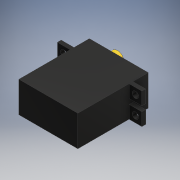
# Autodesk Inventor part: microservo_FT_2322
Saved by Autodesk Inventor 2018 (Build 220112000, 112)
## iProperties
Created: 2018-04-24
Part Number: microservo_FT_2322
Material: Genérico
Document SubType Name: Modeling
Designer: se_ma
Density: 1 g/cm^3
Appearance: Valor por defecto
Author: se_ma
Autodesk Inventor part; units mm, degrees
ref_plane "YZ Plane" through (0, 0, 0) normal (1, 0, 0) x (0, 1, 0)
ref_plane "XZ Plane" through (0, 0, 0) normal (0, 1, 0) x (-1, 0, 0)
ref_plane "XY Plane" through (0, 0, 0) normal (0, 0, 1) x (1, 0, 0)
sketch "Boceto1" plane through (0, 0, 0) normal (0, 1, 0) x (-1, 0, 0)
  line L0 (0, 0) -> (23, 0)
  line L1 (23, 0) -> (23, -12)
  line L2 (23, -12) -> (0, -12)
  line L3 (0, -12) -> (0, 0)
  dimension "d0" = 23
  dimension "d1" = 12
  constraints: 8 end point, 2 parallel, 1 horizontal, 1 perpendicular
  measures "d0" distance of L1.end L2.end
  measures "d1" distance of L0.end L1.end
extrude "Extrusión1" add sketch "Boceto1" along normal blind 27.5
sketch "Boceto2" plane through (0, 27.5, 0) normal (0, 1, 0) x (1, 0, 0)
  line L0 (0, 0) -> (0, 12) projected
  line L1 (0, 0) -> (0, 12)
  line L2 (0, 6) -> (-17, 6)
  circle A0 centre (-17, 6) radius 4.25
  circle A1 centre (-17, 6) radius 2.5
  dimension "d4" = 17
  dimension "d5" = 8.5
  dimension "d6" = 5
  constraints: 4 end point, 2 centre point, 2 coincident, 1 collinear, 1 horizontal, 1 midpoint
  measures "d4" distance of L2.start L2.end
  measures "d5" diameter of A0
  measures "d6" diameter of A1
extrude "Extrusión2" add sketch "Boceto2" along normal blind 5 contours A1
sketch "Boceto3" plane through (0, 27.5, 0) normal (0, 1, 0) x (1, 0, 0)
  circle A0 centre (-17, 6) radius 2.5 projected
  circle A1 centre (-17, 6) radius 4.25
  point P0 (0, 0)
  dimension "d9" = 8.5
  constraints: 1 centre point, 1 coincident
  measures "d9" diameter of A1
extrude "Extrusión3" add sketch "Boceto3" along normal blind 1.5
sketch "Boceto4" plane through (-23, 0, -12) normal (-1, 0, 0) x (0, 0, 1)
  line L0 (12, 0) -> (12, 27.5) projected
  line L1 (12, 27.5) -> (12, 20)
  line L2 (12, 20) -> (12, 21.5)
  line L3 (0, 0) -> (0, 27.5) projected
  line L4 (12, 21.5) -> (7, 21.5)
  line L5 (7, 21.5) -> (7, 20)
  line L6 (7, 20) -> (12, 20)
  line L7 (0, 21.5) -> (5, 21.5)
  line L8 (5, 21.5) -> (5, 20)
  line L9 (5, 20) -> (0, 20)
  line L10 (0, 21.5) -> (0, 20)
  dimension "d12" = 7.5
  dimension "d13" = 1.5
  dimension "d14" = 5
  dimension "d15" = 5
  constraints: 18 end point, 8 point on line, 3 perpendicular, 1 collinear, 1 horizontal
  measures "d12" distance of L0.end L1.end
  measures "d13" distance of L1.end L2.end
  measures "d14" distance of L2.end L4.end
  measures "d15" distance of L7.start L7.end
extrude "Extrusión4" add sketch "Boceto4" along normal blind 5 and the other way blind 28
sketch "Boceto5" plane through (-23, 21.5, -7) normal (0, 1, 0) x (1, 0, 0)
  line L0 (-5, 0) -> (-5, 5) projected
  line L1 (-5, 2.5) -> (0, 2.5)
  line L2 (0, -7) -> (0, 5) projected
  circle A0 centre (-2.5, 2.5) radius 1.25
  circle A1 centre (-2.5, -4.5) radius 1.25
  line L3 (28, 0) -> (28, 5) projected
  line L4 (28, 2.5) -> (23, 2.5)
  circle A2 centre (25.5, 2.5) radius 1.25
  circle A3 centre (25.5, -4.5) radius 1.25
  point P0 (23, -7)
  dimension "d20" = 2.5
  dimension "d21" = 2.5
  dimension "d22" = 2.5
  dimension "d23" = 2.5
  constraints: 4 centre point, 4 end point, 4 midpoint, 2 horizontal, 1 point on line
  measures "d20" diameter of A0
  measures "d21" diameter of A1
  measures "d22" diameter of A2
  measures "d23" diameter of A3
extrude "Extrusión5" cut sketch "Boceto5" against normal blind 5
sketch "Boceto6" plane through (-23, 0, -12) normal (-1, 0, 0) x (0, 0, 1)
  line L0 (12, 0) -> (12, 20) projected
  line L1 (12, 20) -> (12, 9.5)
  line L2 (12, 9.5) -> (0, 9.5)
  line L3 (0, 0) -> (0, 20) projected
  line L4 (6, 9.5) -> (9, 9.5)
  line L5 (9, 9.5) -> (9, 5)
  line L6 (9, 5) -> (3, 5)
  line L7 (3, 5) -> (3, 9.5)
  dimension "d26" = 10.5
  dimension "d27" = 3
  dimension "d28" = 4.5
  dimension "d29" = 6
  constraints: 12 end point, 4 perpendicular, 4 point on line, 1 midpoint
  measures "d26" distance of L0.end L1.end
  measures "d27" distance of L4.start L4.end
  measures "d28" distance of L4.end L5.end
  measures "d29" distance of L5.end L6.end
extrude "Extrusión6" cut sketch "Boceto6" against normal blind 5
